Autodesk Fusion 360 part; units mm, degrees
(part 2 of 2)
sketch "Boceto12" plane through (0, 0, -1.87) normal (0, 0, 1) x (1, 0, 0)
  line L0 (9.07, -36.4925) -> (12.07, -36.4925)
  line L1 (14.57, -38.9925) -> (14.57, -41.9925)
  line L2 (12.07, -44.4925) -> (9.07, -44.4925)
  line L3 (6.57, -41.9925) -> (6.57, -38.9925)
  arc A0 (9.07, -36.4925) -> (6.57, -38.9925) centre (9.07, -38.9925) ccw
  arc A1 (14.57, -38.9925) -> (12.07, -36.4925) centre (12.07, -38.9925) ccw
  arc A2 (12.07, -44.4925) -> (14.57, -41.9925) centre (12.07, -41.9925) ccw
  arc A3 (6.57, -41.9925) -> (9.07, -44.4925) centre (9.07, -41.9925) ccw
  line L4 (-5.025, -46.13) -> (4.975, -46.13)
  line L5 (6.7415, -35.2425) -> (16, -35.2425) construction
  line L6 (6.7415, -35.2425) -> (16, -35.2425) construction
  arc A4 (6.57, -31.4925) -> (9.07, -33.9925) centre (9.07, -31.4925) ccw
  line L7 (9.07, -33.9925) -> (12.07, -33.9925)
  arc A5 (12.07, -33.9925) -> (14.57, -31.4925) centre (12.07, -31.4925) ccw
  line L8 (14.57, -31.4925) -> (14.57, -28.4925)
  arc A6 (14.57, -28.4925) -> (12.07, -25.9925) centre (12.07, -28.4925) ccw
  line L9 (12.07, -25.9925) -> (9.07, -25.9925)
  arc A7 (9.07, -25.9925) -> (6.57, -28.4925) centre (9.07, -28.4925) ccw
  line L10 (6.57, -28.4925) -> (6.57, -31.4925)
  line L11 (-7.545, -22.755) -> (7.545, -22.755)
  line L12 (19.92, -39.73) -> (19.92, -17.225)
  line L13 (21.57, -47.73) -> (-21.57, -47.73) construction
  line L14 (13.52, -47.73) -> (-13.57, -47.73)
  line L15 (21.57, -22.755) -> (21.57, -47.73) construction
  line L16 (21.52, 17.28) -> (21.52, -39.73)
  line L17 (-21.57, -47.73) -> (-21.57, -22.755) construction
  line L18 (-21.57, -22.755) -> (21.57, -22.755) construction
  line L19 (10.57, -25.9925) -> (10.57, -22.755) construction
  line L20 (10.57, -44.4925) -> (10.57, -47.73) construction
  arc A8 (9.07, -36.2925) -> (6.37, -38.9925) centre (9.07, -38.9925) ccw
  line L21 (6.37, -41.9925) -> (6.37, -38.9925)
  arc A9 (6.37, -41.9925) -> (9.07, -44.6925) centre (9.07, -41.9925) ccw
  line L22 (12.07, -44.6925) -> (9.07, -44.6925)
  arc A10 (12.07, -44.6925) -> (14.77, -41.9925) centre (12.07, -41.9925) ccw
  line L23 (14.77, -38.9925) -> (14.77, -41.9925)
  arc A11 (14.77, -38.9925) -> (12.07, -36.2925) centre (12.07, -38.9925) ccw
  line L24 (9.07, -36.2925) -> (12.07, -36.2925)
  arc A12 (6.37, -31.4925) -> (9.07, -34.1925) centre (9.07, -31.4925) ccw
  line L25 (9.07, -34.1925) -> (12.07, -34.1925)
  arc A13 (12.07, -34.1925) -> (14.77, -31.4925) centre (12.07, -31.4925) ccw
  line L26 (14.77, -31.4925) -> (14.77, -28.4925)
  arc A14 (14.77, -28.4925) -> (12.07, -25.7925) centre (12.07, -28.4925) ccw
  line L27 (12.07, -25.7925) -> (9.07, -25.7925)
  arc A15 (9.07, -25.7925) -> (6.37, -28.4925) centre (9.07, -28.4925) ccw
  line L28 (6.37, -28.4925) -> (6.37, -31.4925)
  arc A16 (9.07, -35.4925) -> (5.57, -38.9925) centre (9.07, -38.9925) ccw
  line L29 (5.57, -41.9925) -> (5.57, -38.9925)
  arc A17 (5.57, -41.9925) -> (9.07, -45.4925) centre (9.07, -41.9925) ccw
  line L30 (12.07, -45.4925) -> (9.07, -45.4925)
  arc A18 (12.07, -45.4925) -> (15.57, -41.9925) centre (12.07, -41.9925) ccw
  line L31 (15.57, -38.9925) -> (15.57, -41.9925)
  arc A19 (15.57, -38.9925) -> (12.07, -35.4925) centre (12.07, -38.9925) ccw
  line L32 (9.07, -35.4925) -> (12.07, -35.4925)
  line L33 (5.57, -28.4925) -> (5.57, -31.4925)
  arc A20 (9.07, -24.9925) -> (5.57, -28.4925) centre (9.07, -28.4925) ccw
  line L34 (12.07, -24.9925) -> (9.07, -24.9925)
  arc A21 (15.57, -28.4925) -> (12.07, -24.9925) centre (12.07, -28.4925) ccw
  line L35 (15.57, -31.4925) -> (15.57, -28.4925)
  arc A22 (12.07, -34.9925) -> (15.57, -31.4925) centre (12.07, -31.4925) ccw
  line L36 (9.07, -34.9925) -> (12.07, -34.9925)
  arc A23 (5.57, -31.4925) -> (9.07, -34.9925) centre (9.07, -31.4925) ccw
  arc A24 (-5.57, -27.7425) -> (-8.2776, -25.2511) centre (-8.07, -27.7425) ccw
  arc A25 (-8.2776, -25.2511) -> (-10.57, -27.7425) centre (-8.07, -27.7425) ccw
  arc A26 (-7.9564, -45.2399) -> (-5.57, -42.7425) centre (-8.07, -42.7425) ccw
  arc A27 (-10.57, -42.7425) -> (-7.9564, -45.2399) centre (-8.07, -42.7425) ccw
  arc A28 (1.9238, -35.066) -> (-0.57, -32.7425) centre (-0.57, -35.2425) ccw
  arc A29 (-0.57, -37.7425) -> (1.9238, -35.066) centre (-0.57, -35.2425) ccw
  arc A30 (-15.57, -32.7425) -> (-15.6312, -32.7432) centre (-15.57, -35.2425) ccw
  arc A31 (-15.6312, -32.7432) -> (-15.57, -37.7425) centre (-15.57, -35.2425) ccw
  line L37 (-0.57, -32.7425) -> (-4.07, -32.7425)
  line L38 (-12.07, -32.7425) -> (-15.57, -32.7425)
  line L39 (-5.57, -27.7425) -> (-5.57, -31.2425)
  line L40 (-5.57, -39.2425) -> (-5.57, -42.7425)
  line L41 (-10.57, -31.2425) -> (-10.57, -27.7425)
  line L42 (-10.57, -42.7425) -> (-10.57, -39.2425)
  line L43 (-15.57, -37.7425) -> (-12.07, -37.7425)
  line L44 (-4.07, -37.7425) -> (-0.57, -37.7425)
  line L45 (-8.07, -42.7425) -> (-8.07, -47.73) construction
  line L46 (-8.07, -27.7425) -> (-8.07, -22.755) construction
  arc A32 (-4.07, -37.7425) -> (-5.57, -39.2425) centre (-4.07, -39.2425) ccw
  arc A33 (-5.57, -31.2425) -> (-4.07, -32.7425) centre (-4.07, -31.2425) ccw
  arc A34 (-12.07, -32.7425) -> (-10.57, -31.2425) centre (-12.07, -31.2425) ccw
  arc A35 (-10.57, -39.2425) -> (-12.07, -37.7425) centre (-12.07, -39.2425) ccw
  arc A36 (-10.77, -42.7425) -> (-7.9473, -45.4397) centre (-8.07, -42.7425) ccw
  arc A37 (-7.9473, -45.4397) -> (-5.37, -42.7425) centre (-8.07, -42.7425) ccw
  line L47 (-5.37, -39.2425) -> (-5.37, -42.7425)
  arc A38 (-4.07, -37.9425) -> (-5.37, -39.2425) centre (-4.07, -39.2425) ccw
  line L48 (-4.07, -37.9425) -> (-0.57, -37.9425)
  arc A39 (-0.57, -37.9425) -> (2.1233, -35.0519) centre (-0.57, -35.2425) ccw
  arc A40 (2.1233, -35.0519) -> (-0.57, -32.5425) centre (-0.57, -35.2425) ccw
  line L49 (-0.57, -32.5425) -> (-4.07, -32.5425)
  arc A41 (-5.37, -31.2425) -> (-4.07, -32.5425) centre (-4.07, -31.2425) ccw
  line L50 (-5.37, -27.7425) -> (-5.37, -31.2425)
  arc A42 (-5.37, -27.7425) -> (-8.2942, -25.0518) centre (-8.07, -27.7425) ccw
  arc A43 (-8.2942, -25.0518) -> (-10.77, -27.7425) centre (-8.07, -27.7425) ccw
  line L51 (-10.77, -31.2425) -> (-10.77, -27.7425)
  arc A44 (-12.07, -32.5425) -> (-10.77, -31.2425) centre (-12.07, -31.2425) ccw
  line L52 (-12.07, -32.5425) -> (-15.57, -32.5425)
  arc A45 (-15.57, -32.5425) -> (-15.6361, -32.5433) centre (-15.57, -35.2425) ccw
  arc A46 (-15.6361, -32.5433) -> (-15.57, -37.9425) centre (-15.57, -35.2425) ccw
  line L53 (-15.57, -37.9425) -> (-12.07, -37.9425)
  arc A47 (-10.77, -39.2425) -> (-12.07, -37.9425) centre (-12.07, -39.2425) ccw
  line L54 (-10.77, -42.7425) -> (-10.77, -39.2425)
  arc A48 (-8.344, -24.4539) -> (-11.37, -27.7425) centre (-8.07, -27.7425) ccw
  line L55 (-11.37, -31.2425) -> (-11.37, -27.7425)
  arc A49 (-12.07, -31.9425) -> (-11.37, -31.2425) centre (-12.07, -31.2425) ccw
  line L56 (-12.07, -31.9425) -> (-15.57, -31.9425)
  arc A50 (-15.57, -31.9425) -> (-15.6508, -31.9435) centre (-15.57, -35.2425) ccw
  arc A51 (-15.6508, -31.9435) -> (-15.57, -38.5425) centre (-15.57, -35.2425) ccw
  line L57 (-15.57, -38.5425) -> (-12.07, -38.5425)
  arc A52 (-11.37, -39.2425) -> (-12.07, -38.5425) centre (-12.07, -39.2425) ccw
  line L58 (-11.37, -42.7425) -> (-11.37, -39.2425)
  arc A53 (-11.37, -42.7425) -> (-7.92, -46.0391) centre (-8.07, -42.7425) ccw
  arc A54 (-7.92, -46.0391) -> (-4.77, -42.7425) centre (-8.07, -42.7425) ccw
  line L59 (-4.77, -39.2425) -> (-4.77, -42.7425)
  arc A55 (-4.07, -38.5425) -> (-4.77, -39.2425) centre (-4.07, -39.2425) ccw
  line L60 (-4.07, -38.5425) -> (-0.57, -38.5425)
  arc A56 (-0.57, -38.5425) -> (2.7218, -35.0095) centre (-0.57, -35.2425) ccw
  arc A57 (2.7218, -35.0095) -> (-0.57, -31.9425) centre (-0.57, -35.2425) ccw
  line L61 (-0.57, -31.9425) -> (-4.07, -31.9425)
  arc A58 (-4.77, -31.2425) -> (-4.07, -31.9425) centre (-4.07, -31.2425) ccw
  line L62 (-4.77, -27.7425) -> (-4.77, -31.2425)
  arc A59 (-4.77, -27.7425) -> (-8.344, -24.4539) centre (-8.07, -27.7425) ccw
  circle A60 centre (-16.3126, -26.9999) radius 2
  line L63 (-12.07, -31.2425) -> (-14, -31.2425) construction
  line L64 (-12.07, -31.2425) -> (-16.3126, -26.9999) construction
  circle A61 centre (-16.3126, -26.9999) radius 2.1
  point P0 (6.57, -36.4925)
  point P1 (14.57, -36.4925)
  point P2 (14.57, -44.4925)
  point P3 (-7.5, -33)
  point P4 (-7.5, -33)
  dimension "d153" = 8
  dimension "d154" = 8
  dimension "d155" = 2.5
  dimension "d156" = 2.5
  dimension "d157" = 2.5
  dimension "d158" = 2.5
  dimension "d160" = 1.25
  dimension "d163" = 7
  dimension "d164" = -0.2
  dimension "d165" = -1
  dimension "d194" = 5
  dimension "d195" = 5
  dimension "d196" = 2.5
  dimension "d204" = 15
  dimension "d205" = 15
  dimension "d207" = 6
  dimension "d209" = 1.5
  dimension "d212" = 3.5
  dimension "d213" = -0.2
  dimension "d214" = -0.8
  dimension "d223" = 4
  dimension "d225" = 45
  dimension "d226" = 6
  dimension "d229" = 0.1
  constraint horizontal L0
  constraint vertical L1
  constraint horizontal L2
  constraint vertical L3
  constraint coincident P0 L0
  constraint coincident P0 L3
  constraint tangent L0 A0
  constraint tangent L3 A0
  constraint coincident P1 L0
  constraint coincident P1 L1
  constraint tangent L0 A1
  constraint tangent L1 A1
  constraint coincident P2 L1
  constraint coincident P2 L2
  constraint tangent L1 A2
  constraint tangent L2 A2
  constraint tangent L3 A3
  constraint tangent L2 A3
  constraint parallel L0 L5
  constraint symmetric L0.start L5 A4.end
  constraint symmetric L3.end L5 A4.start
  constraint symmetric A0 L5 A4
  constraint symmetric L0.end L5 L7.end
  constraint symmetric L1.start L5 A5.end
  constraint symmetric A1 L5 A5
  constraint symmetric L1.end L5 L8.end
  constraint symmetric L2.start L5 A6.end
  constraint symmetric A2 L5 A6
  constraint symmetric L3.start L5 A7.end
  constraint symmetric L2.end L5 L9.end
  constraint symmetric A3 L5 A7
  constraint symmetric L6.end L5 L5.end
  constraint horizontal L13
  constraint midpoint L13 L14
  constraint vertical L15
  constraint coincident L13.start L15.end
  constraint coincident L16 L15.start
  constraint perpendicular L13 L17
  constraint perpendicular L16 L18
  constraint midpoint L11 L18
  constraint midpoint L9 L19.start
  constraint coincident L18 L19.end
  constraint perpendicular L18 L19
  constraint midpoint L2 L20.start
  constraint perpendicular L14 L20
  constraint coincident L13 L20.end
  constraint equal L19 L20
  constraint symmetric L6 A8.start A12.end
  constraint symmetric L6 A8.end A12.start
  constraint symmetric L6 A8 A12
  constraint symmetric L6 L21.start A15.end
  constraint symmetric L6 A9.end L27.end
  constraint symmetric L6 A9 A15
  constraint symmetric L6 L22.start A14.end
  constraint symmetric L6 A10.end L26.end
  constraint symmetric L6 A10 A14
  constraint symmetric L6 L23.start A13.end
  constraint symmetric L6 A11.end L25.end
  constraint symmetric L6 A11 A13
  constraint symmetric L5 A16.start L36.start
  constraint symmetric L5 A16.end L33.end
  constraint symmetric L5 A16 A23
  constraint symmetric L5 L29.start L33.start
  constraint symmetric L5 A17.end A20.start
  constraint symmetric L5 A17 A20
  constraint symmetric L5 L30.start L34.start
  constraint symmetric L5 A18.end A21.start
  constraint symmetric L5 A18 A21
  constraint symmetric L5 L31.start L35.start
  constraint symmetric L5 A19.end A22.start
  constraint symmetric L5 A19 A22
  constraint horizontal L43
  constraint coincident P4 P3
  constraint tangent A24 L39
  constraint tangent A25 L42
  constraint coincident A24.end A25.start
  constraint tangent A26 L39
  constraint tangent A27 L42
  constraint coincident A26.start A27.end
  constraint tangent A28 L37
  constraint tangent A29 L43
  constraint coincident A28.start A29.end
  constraint tangent A30 L37
  constraint tangent A31 L43
  constraint coincident A30.end A31.start
  constraint collinear L37 L38
  constraint collinear L39 L40
  constraint collinear L41 L42
  constraint collinear L43 L44
  constraint coincident A26.centre A27.centre
  constraint vertical L45
  constraint coincident L13 L45.end
  constraint coincident A24.centre A25.centre
  constraint perpendicular L11 L46
  constraint coincident L18 L46.end
  constraint equal L45 L46
  constraint tangent L40 A32
  constraint tangent L44 A32
  constraint tangent L37 A33
  constraint tangent L39 A33
  constraint tangent L41 A34
  constraint tangent L38 A34
  constraint tangent L42 A35
  constraint tangent L43 A35
  constraint equal A33 A34
  constraint equal A34 A35
  constraint equal A32 A35
  constraint equal L38 L41
  constraint equal L39 L41
  constraint equal L37 L39
  constraint equal L37 L44
  constraint equal L40 L44
  constraint equal L40 L42
  constraint equal L42 L43
  constraint equal A24 A25
  constraint equal A25 A31
  constraint equal A27 A31
  constraint equal A26 A27
  constraint equal A26 A29
  constraint equal A28 A29
  constraint coincident A34.centre A44.centre
  constraint horizontal L63
  constraint coincident A60.centre L64.end
  measures "d153" distance of P1 P2
  measures "d154" distance of P0 P1
  measures "d155" radius of A0
  measures "d156" radius of A1
  measures "d157" radius of A2
  measures "d158" radius of A3
  measures "d160" distance of L0 L5
  measures "d163" distance of L8 L15
  measures "d194" distance of L37 L43
  measures "d195" distance of L39 L42
  measures "d196" radius of A24
  measures "d204" distance of A24.centre A26.centre
  measures "d205" distance of A28.centre A30.centre
  measures "d207" distance of L17 A30.centre
  measures "d209" radius of A33
  measures "d212" distance of A24.start L39.end
  measures "d223" diameter of A60
  measures "d225" angle of L63 L64
  measures "d226" distance of A34.centre A60.centre
extrude "Extruir16" cut sketch "Boceto12" along normal up to surface (4 mm away) contours L0 L1 L2 L3 A0 A1 A2 A3 | A4 L7 A5 L8 A6 L9 A7 L10 | A8 L21 A9 L22 A10 L23 A11 L24 | A12 L25 A13 L26 A14 L27 A15 L28 bodies 7 6 8 9 4
extrude "Extruir17" add sketch "Boceto12" along normal up to surface (5 mm away) separate body contours L0 L1 L2 L3 A0 A1 A2 A3 | A4 L7 A5 L8 A6 L9 A7 L10 makes body 16 at (11.07, -41.8258, -1.87) makes body 17 at (10.07, -28.6592, -1.87)
extrude "Extruir18" add sketch "Boceto12" along normal up to surface (2 mm away) separate body contours A8 L21 A9 L22 A10 L23 A11 L24 | A12 L25 A13 L26 A14 L27 A15 L28 | A16 L29 A17 L30 A18 L31 A19 L32 | L33 A20 L34 A21 L35 A22 L36 A23 makes body 18 at (11.07, -34.3258, -1.87) makes body 19 at (5.9033, -39.9925, -1.87)
combine "Combinar7" operation add target body 16 tool bodies 19
combine "Combinar8" operation add target body 17 tool bodies 18
sketch "Boceto13" plane through (0, 0, 3.13) normal (0, 0, 1) x (-1, 0, 0)
  arc A0 (-9.07, 25.9925) -> (-6.57, 28.4925) centre (-9.07, 28.4925) ccw
  line L0 (-6.57, 28.4925) -> (-6.57, 31.4925)
  arc A1 (-6.57, 31.4925) -> (-9.07, 33.9925) centre (-9.07, 31.4925) ccw
  line L1 (-9.07, 33.9925) -> (-12.07, 33.9925)
  arc A2 (-12.07, 33.9925) -> (-14.57, 31.4925) centre (-12.07, 31.4925) ccw
  line L2 (-14.57, 31.4925) -> (-14.57, 28.4925)
  arc A3 (-14.57, 28.4925) -> (-12.07, 25.9925) centre (-12.07, 28.4925) ccw
  line L3 (-12.07, 25.9925) -> (-9.07, 25.9925)
  line L4 (-6.57, 26.2188) -> (-6.57, 33.7662) construction
  line L5 (-6.57, 36.6984) -> (-6.57, 44.2866) construction
  line L6 (-6.57, 41.9925) -> (-6.57, 38.9925)
  line L7 (-14.57, 26.1781) -> (-14.57, 33.8069) construction
  line L8 (-14.57, 36.6781) -> (-14.57, 44.3069) construction
  line L9 (-14.57, 38.9925) -> (-14.57, 41.9925)
  line L10 (-14.57, 40.4925) -> (-6.57, 40.4925) construction
  line L11 (-6.57, 29.9925) -> (-14.57, 29.9925) construction
  circle A4 centre (-10.57, 29.9925) radius 3
  circle A5 centre (-10.57, 40.4925) radius 3
  dimension "d172" = 6
  constraint vertical L4
  constraint midpoint L0 L4
  constraint vertical L5
  constraint midpoint L5 L6
  constraint vertical L7
  constraint midpoint L2 L7
  constraint vertical L8
  constraint midpoint L8 L9
  constraint midpoint L9 L10.start
  constraint midpoint L6 L10.end
  constraint midpoint L0 L11.start
  constraint midpoint L2 L11.end
  constraint midpoint L11 A4.centre
  constraint midpoint L10 A5.centre
  constraint equal A4 A5
  measures "d172" diameter of A4
extrude "Extruir19" add sketch "Boceto13" along normal blind 1 contours A4 | A5 bodies 16 17
fillet "Empalme8" radius 0.2 2 edges at (13.367, -39.4077, 4.13) (13.367, -28.9077, 4.13) on bodies 16 17
extrude "Extruir20" cut sketch "Boceto12" along normal up to surface (4 mm away) contours A24 A25 A26 A27 A28 A29 A30 A31 L37 L38 L39 L40 L41 L42 L43 L44 A32 A33 A34 A35 | A36 A37 L47 A38 L48 A39 A40 L49 A41 L50 A42 A43 L51 A44 L52 A45 A46 L53 A47 L54 bodies 8 4 9 7 6
extrude "Extruir21" add sketch "Boceto12" along normal up to surface (6 mm away) separate body contours A24 A25 A26 A27 A28 A29 A30 A31 L37 L38 L39 L40 L41 L42 L43 L44 A32 A33 A34 A35 makes body 20
extrude "Extruir22" add sketch "Boceto12" along normal up to surface (2 mm away) separate body contours A36 A37 L47 A38 L48 A39 A40 L49 A41 L50 A42 A43 L51 A44 L52 A45 A46 L53 A47 L54 | A48 L55 A49 L56 A50 A51 L57 A52 L58 A53 A54 L59 A55 L60 A56 A57 L61 A58 L62 A59 makes body 21
combine "Combinar9" operation add target body 20 tool bodies 21
fillet "Empalme9" radius 0.2 32 edges at (-5.57, -40.9925, 4.13) (-8.07, -45.2425, 4.13) (-10.57, -40.9925, 4.13) (-11.0093, -38.1818, 4.13) (-13.82, -37.7425, 4.13) (-18.07, -35.2425, 4.13) (-13.82, -32.7425, 4.13) (-11.0093, -32.3032, 4.13) (-10.57, -29.4925, 4.13) (-8.07, -25.2425, 4.13) (-5.57, -29.4925, 4.13) (-5.1307, -32.3032, 4.13) (-2.32, -32.7425, 4.13) (1.93, -35.2425, 4.13) (-2.32, -37.7425, 4.13) (-5.1307, -38.1818, 4.13) (1.93, -35.2425, 4.13) (-2.32, -37.7425, 4.13) (-5.1307, -38.1818, 4.13) (-5.57, -40.9925, 4.13) (-8.07, -45.2425, 4.13) (-10.57, -40.9925, 4.13) (-11.0093, -38.1818, 4.13) (-13.82, -37.7425, 4.13) (-18.07, -35.2425, 4.13) (-13.82, -32.7425, 4.13) (-11.0093, -32.3032, 4.13) (-10.57, -29.4925, 4.13) (-8.07, -25.2425, 4.13) (-5.57, -29.4925, 4.13) (-5.1307, -32.3032, 4.13) (-2.32, -32.7425, 4.13) on bodies 20
extrude "Extruir24" cut sketch "Boceto12" along normal up to surface (4 mm away) contours A60 | A61 bodies 4 9 8 6 7
extrude "Extruir25" add sketch "Boceto12" along normal up to surface (4 mm away) separate body contours A60 makes body 22
combine "Combinar11" operation add target body 6 tool bodies 4 7 8 9
combine "Combinar12" operation add target body 5 tool bodies 6
sketch "Boceto15" plane through (0, 0, -10.35) normal (0, 0, 1) x (-1, 0, 0)
  circle A0 centre (15.57, 41.73) radius 1.3
  circle A1 centre (-15.52, 41.73) radius 1.3
  circle A2 centre (15.57, -19.28) radius 1.3
  circle A3 centre (-15.52, -19.28) radius 1.3
  line L0 (19.97, 5.225) -> (17.97, 5.225)
  line L1 (17.97, 5.225) -> (17.97, 17.225)
  line L2 (17.97, 17.225) -> (19.97, 17.225)
  line L3 (19.97, 17.225) -> (19.97, 39.73)
  arc A4 (19.97, 39.73) -> (13.57, 46.13) centre (13.57, 39.73) ccw
  line L4 (13.57, 46.13) -> (6.025, 46.13)
  line L5 (6.025, 46.13) -> (6.025, 44.13)
  line L6 (6.025, 44.13) -> (-5.975, 44.13)
  line L7 (-5.975, 44.13) -> (-5.975, 46.13)
  line L8 (-5.975, 46.13) -> (-13.52, 46.13)
  arc A5 (-13.52, 46.13) -> (-19.92, 39.73) centre (-13.52, 39.73) ccw
  line L9 (-19.92, 39.73) -> (-19.92, 17.225)
  line L10 (-19.92, 17.225) -> (-17.92, 17.225)
  line L11 (-17.92, 17.225) -> (-17.92, 5.225)
  line L12 (-17.92, 5.225) -> (-19.92, 5.225)
  line L13 (-19.92, 5.225) -> (-19.92, -17.28)
  arc A6 (-19.92, -17.28) -> (-13.52, -23.68) centre (-13.52, -17.28) ccw
  line L14 (-13.52, -23.68) -> (-5.975, -23.68)
  line L15 (-5.975, -23.68) -> (-5.975, -21.68)
  line L16 (-5.975, -21.68) -> (6.025, -21.68)
  line L17 (6.025, -21.68) -> (6.025, -23.68)
  line L18 (6.025, -23.68) -> (13.57, -23.68)
  arc A7 (13.57, -23.68) -> (19.97, -17.28) centre (13.57, -17.28) ccw
  line L19 (19.97, -17.28) -> (19.97, 5.225)
  line L20 (0.025, 44.13) -> (0.025, -21.68) construction
  line L21 (-14.975, 36.225) -> (15.025, 36.225)
  line L22 (15.025, 36.225) -> (15.025, -13.775)
  line L23 (15.025, -13.775) -> (-14.975, -13.775)
  line L24 (-14.975, -13.775) -> (-14.975, 36.225)
  line L25 (-14.975, 36.225) -> (15.025, -13.775) construction
  line L26 (15.025, 36.225) -> (-14.975, -13.775) construction
  point P0 (0.025, 11.225)
  dimension "d235" = 30
  dimension "d236" = 50
  constraint midpoint L6 L20.start
  constraint midpoint L16 L20.end
  constraint horizontal L21
  constraint perpendicular L21 L22
  constraint parallel L21 L23
  constraint parallel L22 L24
  constraint coincident L25 P0
  constraint coincident L26 P0
  constraint midpoint L20 P0
  measures "d235" distance of L22.end L23.end
  measures "d236" distance of L21.start L23.end
extrude "Extruir26" cut sketch "Boceto15" against normal up to surface (1.52 mm away) contours L21 L22 L23 L24 bodies 10
fillet "Empalme10" radius 2 4 edges at (14.975, 13.775, -11.11) (-15.025, 13.775, -11.11) (-15.025, -36.225, -11.11) (14.975, -36.225, -11.11) on bodies 10
equation "d61 = 11.5 mm + 0.05 mm"
equation "d68 = 38.14 mm + 0.1 mm"
equation "d107 = -1.72 mm - 0.8 mm"
named bodies: "Display", "Marco", "Cristal", "Carcasa", "Tapa", "PCB", "BotDown", "BotUp", "Cruz", "LED"
